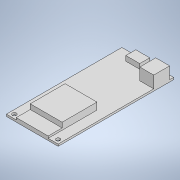
# Autodesk Inventor part: ESP32 LOLIN32 V1.0.0
Saved by Autodesk Inventor 2020 (Build 240168000, 168)
## iProperties
Created: 2021-08-09
Part Number: ESP32 LOLIN32 V1.0.0
Material: Типовые
Document SubType Name: Modeling
Designer: Антон
Density: 1 g/cm^3
Appearance: По умолчанию
Author: Антон
Autodesk Inventor part; units mm, degrees
ref_plane "YZ Plane" through (0, 0, 0) normal (1, 0, 0) x (0, 1, 0)
ref_plane "XZ Plane" through (0, 0, 0) normal (0, 1, 0) x (-1, 0, 0)
ref_plane "XY Plane" through (0, 0, 0) normal (0, 0, 1) x (1, 0, 0)
sketch "Эскиз1" plane through (0, 0, 0) normal (0, 1, 0) x (-1, 0, 0)
  line L0 (0, 0) -> (26, 0)
  line L1 (26, 0) -> (26, -58)
  line L2 (26, -58) -> (0, -58)
  line L3 (0, -58) -> (0, 0)
  dimension "d0" = 58
  dimension "d1" = 26
  constraints: 8 end point, 2 parallel, 1 horizontal, 1 perpendicular
  measures "d0" distance of L0.end L1.end
  measures "d1" distance of L1.end L2.end
extrude "Выдавливание1" add sketch "Эскиз1" along normal blind 1
sketch "Эскиз2" plane through (0, 1, 0) normal (0, 1, 0) x (1, 0, 0)
  line L0 (-26, 0) -> (0, 0) projected
  line L1 (-26, 58) -> (-26, 0) projected
  line L2 (0, 0) -> (0, 58) projected
  point P0 (-24, 2)
  point P1 (-2, 2)
  dimension "d4" = 2
  dimension "d5" = 2
  dimension "d6" = 2
  dimension "d7" = 2
  measures "d4" distance from line of L0 point (-24, 2)
  measures "d5" distance from line of L1 point (-24, 2)
  measures "d6" distance from line of L2 point (-2, 2)
  measures "d7" distance from line of L0 point (-2, 2)
hole "Отверстие1" at (-24, 1, -2) at (-2, 1, -2) direction (0, -1, 0) diameter 2 end through all
sketch "Эскиз3" plane through (0, 1, 0) normal (0, 1, 0) x (1, 0, 0)
  line L0 (-12, 53) -> (-19, 53)
  line L1 (-19, 53) -> (-19, 58)
  line L2 (-19, 58) -> (-12, 58)
  line L3 (-12, 58) -> (-12, 53)
  line L4 (0, 58) -> (-26, 58) projected
  line L5 (-26, 58) -> (-26, 0) projected
  point P0 (0, 0)
  dimension "d15" = 7
  dimension "d16" = 5
  dimension "d17" = 7
  constraints: 8 end point, 2 parallel, 1 collinear, 1 horizontal, 1 perpendicular
  measures "d15" distance of L1.end L2.end
  measures "d16" distance of L0.end L1.end
  measures "d17" distance between parallel lines of L5 L1
extrude "Выдавливание2" add sketch "Эскиз3" along normal blind 2.5
sketch "Эскиз4" plane through (0, 1, 0) normal (0, 1, 0) x (1, 0, 0)
  line L0 (-7, 48) -> (0, 48)
  line L1 (0, 48) -> (0, 56)
  line L2 (0, 56) -> (-7, 56)
  line L3 (-7, 56) -> (-7, 48)
  line L4 (0, 0) -> (0, 58) projected
  line L5 (0, 58) -> (-12, 58) projected
  dimension "d20" = 7
  dimension "d21" = 8
  dimension "d22" = 2
  constraints: 8 end point, 2 parallel, 1 collinear, 1 horizontal, 1 perpendicular
  measures "d20" distance of L2.end L1.end
  measures "d21" distance of L1.end L0.end
  measures "d22" distance between parallel lines of L5 L2
extrude "Выдавливание3" add sketch "Эскиз4" along normal blind 6
sketch "Эскиз5" plane through (0, 1, 0) normal (0, 1, 0) x (1, 0, 0)
  line L0 (-21, 7) -> (-5, 7)
  line L1 (-5, 7) -> (-5, 24.5)
  line L2 (-5, 24.5) -> (-21, 24.5)
  line L3 (-21, 24.5) -> (-21, 7)
  line L4 (-26, 0) -> (0, 0) projected
  point P0 (-13, 7)
  point P1 (-13, 0)
  dimension "d25" = 17.5
  dimension "d26" = 16
  dimension "d27" = 7
  constraints: 8 end point, 2 midpoint, 2 parallel, 1 horizontal, 1 perpendicular, 1 vertical alignment
  measures "d25" distance of L2.end L0.start
  measures "d26" distance of L1.end L2.end
  measures "d27" distance between parallel lines of L4 L0
extrude "Выдавливание4" add sketch "Эскиз5" along normal blind 3.5
sketch "Эскиз6" plane through (0, 1, 0) normal (0, 1, 0) x (1, 0, 0)
  line L0 (-5, 7) -> (-21, 7) projected
  line L1 (-5, 7) -> (-21, 7)
  line L2 (-21, 7) -> (-21, 0)
  line L3 (-21, 0) -> (-5, 0)
  line L4 (-5, 0) -> (-5, 7)
  line L5 (-21, 24.5) -> (-21, 7) projected
  line L6 (-26, 0) -> (0, 0) projected
  constraints: 8 end point, 2 collinear, 2 parallel, 1 horizontal, 1 perpendicular
extrude "Выдавливание5" add sketch "Эскиз6" along normal blind 1
